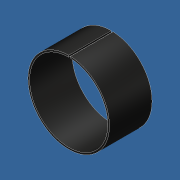
# Autodesk Inventor part: Buffer Piece
Saved by Autodesk Inventor 2018 (Build 220112000, 112)
## iProperties
Created: 2018-02-14
Part Number: Buffer Piece
Material: LCP Plastic
Document SubType Name: Modeling
Designer: Cole
Density: 1.626 g/cm^3
Appearance: Glossy - Black
Author: Cole
Autodesk Inventor part; units mm, degrees
ref_plane "YZ Plane" through (0, 0, 0) normal (1, 0, 0) x (0, 1, 0)
ref_plane "XZ Plane" through (0, 0, 0) normal (0, 1, 0) x (-1, 0, 0)
ref_plane "XY Plane" through (0, 0, 0) normal (0, 0, 1) x (1, 0, 0)
sketch "Sketch1" plane through (0, 0, 0) normal (0, 0, 1) x (1, 0, 0)
  circle A0 centre (0, 0) radius 17.4625
  circle A1 centre (0, 0) radius 18.2245
  dimension "d0" = 34.925
  dimension "d1" = 36.449
  constraints: 2 centre point, 2 coincident
  measures "d0" diameter of A0
  measures "d1" diameter of A1
extrude "Extrusion1" add sketch "Sketch1" along normal blind 19.05
sketch "Sketch2" plane through (0, 0, 19.05) normal (0, 0, 1) x (1, 0, 0)
  circle A0 centre (0, 0) radius 18.2245 projected
  line L0 (0, 18.2245) -> (0, 17.4625)
  circle A1 centre (0, 0) radius 17.4625 projected
  line L1 (0.7937, 18.2072) -> (0.7937, 17.4445)
  dimension "d4" = 0.7937
  constraints: 4 end point, 4 point on circle, 2 vertical, 1 line through centre
  measures "d4" distance between parallel lines of L1 L0
extrude "Extrusion2" cut sketch "Sketch2" against normal blind 19.05 contours L1 A1 L0 A0 picked at (0.7055, 17.702)
body "Solid1"
